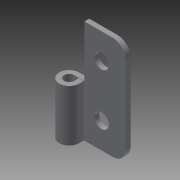
# Autodesk Inventor part: 2838_right
Saved by Autodesk Inventor 2014 SP2 (Build 180246200, 246)
## iProperties
Created: 2018-07-20
Part Number: 2838_right
Material: Generic
Catalog Web Link: www.cadenas.de
Description: 2830, 2831, 2832, 2833, 2835, 2836, 2837, 2838, 2839, 2840, 2841, 2842, 2830-Black, 2831-Black, 2832-Black, 2833-Black, 2835-Black, 2836-Black, 2837-Black, 2838-Black, 2839-Black, 2840-Black, 2841-Black, 2842-Black_right-Economy Lift-Off Hinges
Vendor: 8020
Document SubType Name: Modeling
Designer: psadmin
Manufacturer: 8020
Mass: 3.6839 g
Surface Area: 36.6433 cm^2
Volume: 3.6839 cm^3
Density: 1 g/cm^3
Appearance: PSOLRGB-191-191-191
Category: PARTsolutions
Company: 8020
Title: 2838_right
Author: Cadenas PARTsolutions
Comments: Economy Lift-Off Hinges
PSOL_IDENT_0: {$CADENAS_DATA\23d-libs\8020\inch\panels_and_doors\2830_right.prj},385 {VTYP=3D},{NB=2838_right},{LI
PSOL_IDENT_1: NA=2838_right},{NN=2830, 2831, 2832, 2833, 2835, 2836, 2837, 2838, 2839, 2840, 2841, 2842, 2830-Blac
PSOL_IDENT_2: k, 2831-Black, 2832-Black, 2833-Black, 2835-Black, 2836-Black, 2837-Black, 2838-Black, 2839-Black, 2
PSOL_IDENT_3: 840-Black, 2841-Black, 2842-Black_right},{DATE=16.03.2018 08:23:49},{GEOMDATE=20.11.2017 20:29:52},{
PSOL_IDENT_4: VERSION=},{LINEID=10},{WBVAR=TYPE,FINISH},{WBNUMERIC=}  {NB=2838_right},{LINA=2838_right},{KT=DUMMY}
PSOL_IDENT_5: ,{PN=2838},{SERIES=10 Series},{TYPE=5},{MAT=Aluminum},{FINISH=CA},{A=2.000},{B=1.000},{C=1.000},{D=0
PSOL_IDENT_6: .531},{E=0.281},{F=0.500},{G=0.195},{H=0.187},{J=0.093},{K=0.062},{CAP=40},{R=0.381},{P=0.009},{NO=8
PSOL_IDENT_7: },{CLR=.75,.75,.75}
NN: 2830, 2831, 2832, 2833, 2835, 2836, 2837, 2838, 2839, 2840, 2841, 2842, 2830-Black, 2831-Black, 2832-Black, 2833-Black, 2835-Black, 2836-Black, 2837-Black, 2838-Black, 2839-Black, 2840-Black, 2841-Black, 2842-Black_right
NT: Economy Lift-Off Hinges
NB: 2838_right
NBSYN: $PN._right
LINA: 2838_right
PN: 2838
SERIES: 10 Series
TYPE: Right Hinge Long Pin
MAT: Aluminum
FINISH: Clear Anodize
A: 2
B: 1
C: 1
D: 0.531
E: 0.281
F: 0.5
G: 0.195
H: 0.187
J: 0.093
K: 0.062
CAP: 40
R: 0.381
SUPPLIER: 8020
ARTICLENO: 2838_right
BOMINFO: 2838_right
CREATOR: CADENAS GmbH
Autodesk Inventor part; units mm, degrees
sketch "Sketch_1" plane through (0, 0, 0) normal (0, 1, 0) x (-1, 0, 0)
  arc A0 (0, 0) -> (-4.8387, 4.8387) centre (0, 4.8387) ccw
  line L0 (-4.8387, 4.8387) -> (-4.8387, 2.5527)
  line L1 (-4.8387, 2.5527) -> (-2.4765, 2.5527)
  line L2 (-2.4765, 2.5527) -> (-2.4765, 4.8387)
  arc A1 (0, 2.3622) -> (-2.4765, 4.8387) centre (0, 4.8387) ccw
  line L3 (0, 2.3622) -> (-25.4, 2.3622)
  line L4 (-25.4, 2.3622) -> (-25.4, 0)
  line L5 (-25.4, 0) -> (0, 0)
  constraints: 12 end point, 4 point on circle, 2 centre point
extrude "Extrusion1" add sketch "Sketch_1" along normal mid plane 50.8
sketch "Sketch_2" plane through (0, 0, 0) normal (0, 0, 1) x (1, 0, 0)
  line L0 (-25.4, 50.8) -> (-25.4, -50.8)
  line L1 (-25.4, -50.8) -> (50.8, -50.8)
  line L2 (50.8, -50.8) -> (50.8, 50.8)
  line L3 (50.8, 50.8) -> (-25.4, 50.8)
  line L4 (-12.7, -0.0254) -> (-12.7, -25.4)
  line L5 (-12.7, -25.4) -> (19.05, -25.4)
  arc A0 (19.05, -25.4) -> (25.4, -19.05) centre (19.05, -19.05) ccw
  line L6 (25.4, -19.05) -> (25.4, 19.05)
  arc A1 (25.4, 19.05) -> (19.05, 25.4) centre (19.05, 19.05) ccw
  line L7 (19.05, 25.4) -> (5.0673, 25.4)
  line L8 (5.0673, 25.4) -> (5.0673, -0.0254)
  line L9 (5.0673, -0.0254) -> (-12.7, -0.0254)
  constraints: 20 end point, 4 point on circle, 2 centre point
extrude "Extrusion2" cut sketch "Sketch_2" along normal mid plane 25.4
sketch "Sketch_4" plane through (0, 0, 0) normal (0, 0, 1) x (1, 0, 0)
  circle A0 centre (13.4874, 12.7) radius 3.5687
  constraints: 1 centre point
extrude "Extrusion3" cut sketch "Sketch_4" along normal mid plane 4.7244
sketch "Sketch_5" plane through (0, 0, 0) normal (0, 0, 1) x (1, 0, 0)
  circle A0 centre (13.4874, -12.7) radius 3.5687
  constraints: 1 centre point
extrude "Extrusion4" cut sketch "Sketch_5" along normal mid plane 4.7244
ref_plane "to_left_XY" through (0, 0, 4.8387) normal (0, 1, 0) x (1, 0, 0)
ref_plane "to_left_YZ" through (0, 0, 4.8387) normal (1, 0, 0) x (0, 0, -1)
ref_plane "to_left_ZX" through (0, 0, 4.8387) normal (0, 0, -1) x (0, 1, 0)
body "Solid1"
